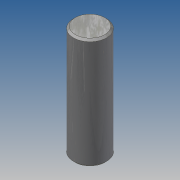
# Autodesk Inventor part: Kolbenbolzen_ra8846s
Saved by Autodesk Inventor 2021 (Build 250183000, 183)
## iProperties
Created: 2020-11-16
Part Number: Kolbenbolzen_ra8846s
Material: Stahl, unlegiert
Document SubType Name: Modeling
Designer: Ricardo A
Density: 7.85 g/cm^3
Appearance: Stahl
Description: Motor_teil_1_kolb.
Mass: 0.955419 g
Surface Area: 1.5332 cm^2
Volume: 0.121709 cm^3
Author: Ricardo A
Revision Number: Rev00
Title: Kolbenzolzen
Subject: Modellmotor
Autodesk Inventor part; units mm, degrees
ref_plane "YZ-Ebene" through (0, 0, 0) normal (1, 0, 0) x (0, 1, 0)
ref_plane "XZ-Ebene" through (0, 0, 0) normal (0, 1, 0) x (-1, 0, 0)
ref_plane "XY-Ebene" through (0, 0, 0) normal (0, 0, 1) x (1, 0, 0)
sketch "Skizze1" plane through (0, 0, 0) normal (0, 0, 1) x (1, 0, 0)
  line L0 (-2.52, 0) -> (2.52, 0) projected
  line L1 (0, -2.52) -> (0, 2.52) projected
  circle A0 centre (0, 0) radius 1.8
  dimension "d0" = 3.6
  constraints: 1 centre point, 1 coincident
  measures "d0" diameter of A0
extrude "Extrusion1" add sketch "Skizze1" along normal blind 12
chamfer "Fase1" distance 0.2 angle 45 2 edges at (-1.8, 0, 12) (-1.8, 0, 0)
